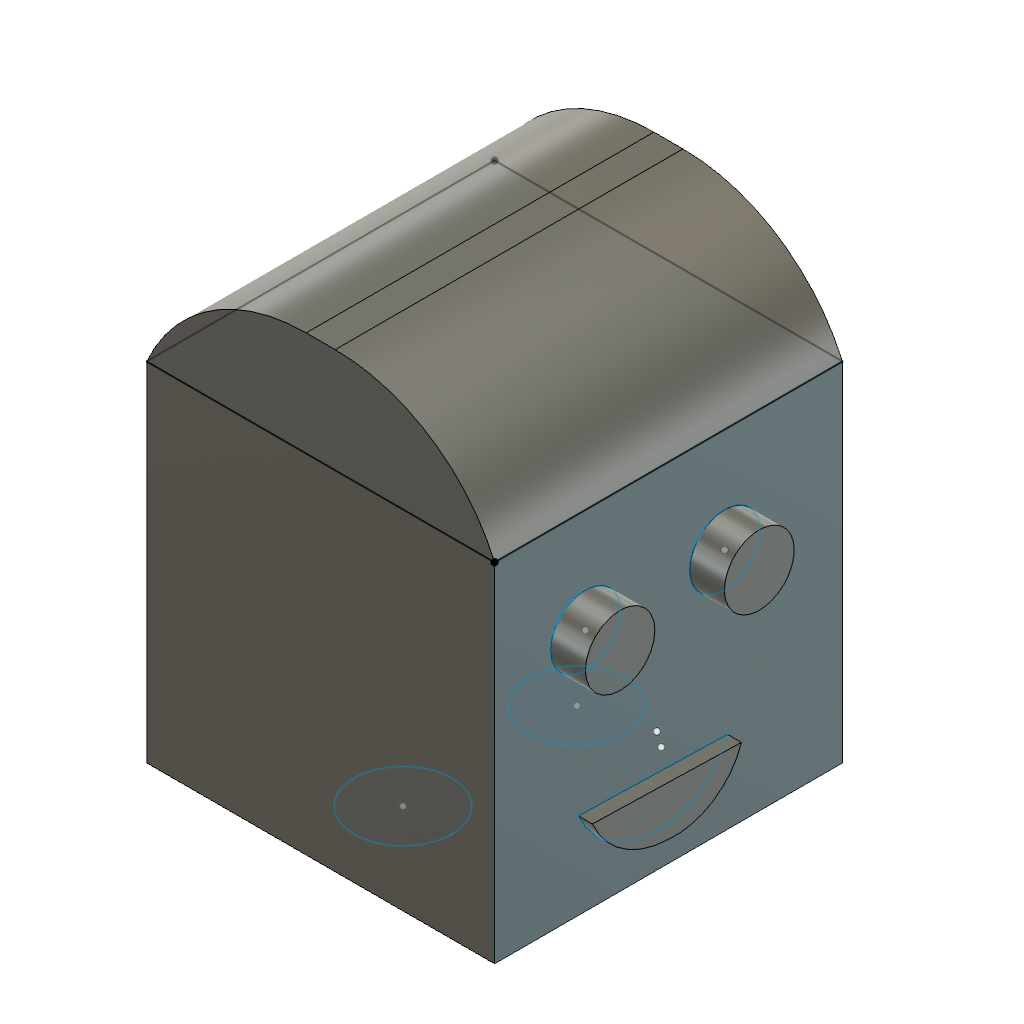
TalkingMinions (Autodesk Fusion 360 design; units mm, degrees)
part number: 2026-09-04-20-08-06-782
Autodesk Fusion 360 part; units mm, degrees
sketch "草图1" plane through (0, 0, 0) normal (0, 0, 1) x (1, 0, 0)
sketch "草图2" plane through (0, 0, 0) normal (0, 1, 0) x (1, 0, 0)
  line L0 (-24.6639, 27.9241) -> (25.3361, 27.9241)
  line L1 (25.3361, 27.9241) -> (25.3361, -22.0759)
  line L2 (25.3361, -22.0759) -> (-24.6639, -22.0759)
  line L3 (-24.6639, -22.0759) -> (-24.6639, 27.9241)
  circle A0 centre (89.9803, -2.0759) radius 60
  dimension "d14" = 50
  dimension "d15" = 50
  dimension "d16" = 30
  dimension "d17" = 120
  constraint horizontal L0
  constraint vertical L1
  constraint horizontal L2
  constraint vertical L3
  measures "d14" distance of L0.end L1.end
  measures "d15" distance of L0.start L0.end
  measures "d16" distance of L0 A0.centre
  measures "d17" diameter of A0
sketch "草图3" plane through (0, 0, 0) normal (0, 1, 0) x (1, 0, 0)
  line L0 (-28.7858, 26.9528) -> (21.2142, 26.9528)
  line L1 (21.2142, 26.9528) -> (21.2142, -23.0472)
  line L2 (21.2142, -23.0472) -> (-28.7858, -23.0472)
  line L3 (-28.7858, -23.0472) -> (-28.7858, 26.9528)
  circle A0 centre (60, 10) radius 30
  dimension "d20" = 50
  dimension "d21" = 50
  dimension "d22" = 60
  constraint horizontal L0
  constraint vertical L1
  constraint horizontal L2
  constraint vertical L3
  measures "d20" distance of L0.start L0.end
  measures "d21" distance of L0.start L2.end
  measures "d22" diameter of A0
extrude "拉伸2" add sketch "草图3" along normal blind 50 contours L0 L1 L2 L3 makes body 1
extrude "拉伸3" add sketch "草图3" along normal blind 30 separate body contours A0 makes body 2
sketch "草图4" plane through (21.2142, 0, 0) normal (1, 0, 0) x (0, 0, -1)
  line L0 (-23.0472, 0) -> (26.9528, 0)
  line L1 (26.9528, 0) -> (26.9528, 50)
  line L2 (26.9528, 50) -> (-23.0472, 50)
  line L3 (-23.0472, 50) -> (-23.0472, 0)
  circle A0 centre (-10, 35) radius 5
  circle A1 centre (10, 35) radius 5
  arc A2 (-10.9914, 12.3886) -> (0, 5) centre (0.2729, 17.2757) ccw
  arc A3 (0, 5) -> (10.4325, 11.8297) centre (0.8975, 15.0118) ccw
  line L4 (-10.9914, 12.3886) -> (10.4325, 11.8297)
  dimension "d27" = 10
  dimension "d28" = 10
  measures "d27" diameter of A0
  measures "d28" diameter of A1
extrude "拉伸4" add sketch "草图4" along normal blind 5 contours A0 bodies 1
extrude "拉伸5" add sketch "草图4" along normal blind 5 contours A1 bodies 1
extrude "拉伸6" add sketch "草图4" along normal blind 2 contours A2 A3 L4 bodies 1
form "造型1" [no effect]
extrude "拉伸7" add 1 faces at (26.2142, 32.8948, 8.6318) along direction (1, 0, 0) blind 5 on bodies 1 bodies 1
extrude "拉伸8" add 1 faces at (26.2142, 31.2655, -9.9692) along direction (1, 0, 0) blind 5 on bodies 1 bodies 1
sketch "草图5" plane through (0, 50, 0) normal (0, 1, 0) x (-1, 0, 0)
  line L0 (28.7858, 23.0472) -> (-21.2142, 23.0472)
  line L1 (-21.2142, 23.0472) -> (-21.2142, -26.9528)
  line L2 (-21.2142, -26.9528) -> (28.7858, -26.9528)
  line L3 (28.7858, -26.9528) -> (28.7858, 23.0472)
  line L4 (-21.2142, 23.0472) -> (28.7858, 23.0472)
  line L5 (28.7858, 23.0472) -> (28.7858, -26.9528)
  line L6 (28.7858, -26.9528) -> (-21.2142, -26.9528)
  line L7 (-21.2142, -26.9528) -> (-21.2142, 23.0472)
  constraint horizontal L4
  constraint vertical L5
  constraint horizontal L6
  constraint vertical L7
  constraint coincident L2.end L3.start
  constraint coincident L0.end L1.start
extrude "拉伸9" add 1 faces at (-12.1191, 50, -10.2861) along direction (0, 1, 0) blind 15 separate body on bodies 1 makes body 3
fillet "圆角1" radius 25 1 edges at (21.2142, 65, -1.9528) on bodies 3
fillet "圆角2" radius 25 1 edges at (-28.7858, 65, -1.9528) on bodies 3
extrude "拉伸10" cut 1 faces at (31.2142, 31.2655, -9.9692) along direction (-1, 0, 0) blind 60 on bodies 1 bodies 1
extrude "拉伸11" cut 1 faces at (31.2142, 32.8948, 8.6318) along direction (-1, 0, 0) blind 5 on bodies 1 bodies 1
extrude "拉伸12" add sketch "草图4" along normal blind 5 separate body contours A1 makes body 4
sketch "草图6" plane through (0, 0, 0) normal (0, 1, 0) x (1, 0, 0)
  circle A0 centre (-5, 15) radius 7
  circle A1 centre (-5, -10) radius 7
  dimension "d51" = 14
  dimension "d52" = 14
  measures "d51" diameter of A0
  measures "d52" diameter of A1
extrude "拉伸13" cut sketch "草图6" along normal blind 2 contours A0 bodies 1
hidden bodies 2
named bodies: "立方体", "圆珠"
